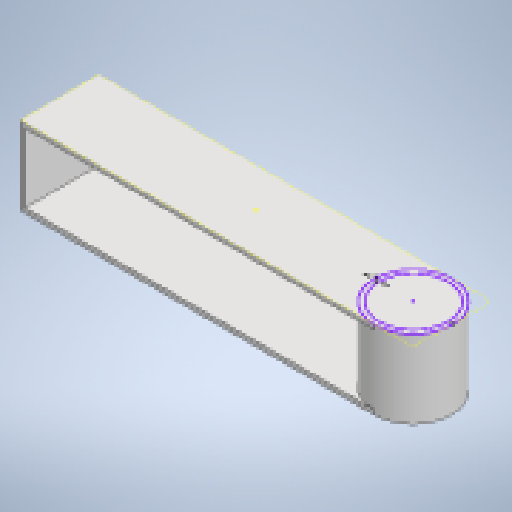
# Autodesk Inventor part: Base_box
Saved by Autodesk Inventor 2023 (Build 270158000, 158)
## iProperties
Created: 2022-04-08
Part Number: Base_box
Material: 一般
Document SubType Name: Modeling
Designer: device
Density: 1 g/cm^3
Appearance: 預設
Author: device
Autodesk Inventor part; units mm, degrees
ref_plane "YZ Plane" through (0, 0, 0) normal (1, 0, 0) x (0, 1, 0)
ref_plane "XZ Plane" through (0, 0, 0) normal (0, 1, 0) x (-1, 0, 0)
ref_plane "XY Plane" through (0, 0, 0) normal (0, 0, 1) x (1, 0, 0)
sketch "草圖1" plane through (0, 0, 0) normal (0, 1, 0) x (-1, 0, 0)
  line L0 (125, 25) -> (-125, 25)
  line L1 (-125, 25) -> (-125, -25)
  line L2 (-125, -25) -> (125, -25)
  line L3 (125, -25) -> (125, 25)
  line L4 (125, 25) -> (-125, -25) construction
  line L5 (-125, 25) -> (125, -25) construction
  point P0 (0, 0)
  dimension "d0" = 250
  dimension "d1" = 50
  constraints: 12 end point, 2 midpoint, 2 parallel, 1 horizontal, 1 perpendicular
  measures "d0" distance of L1.end L2.end
  measures "d1" distance of L0.end L1.end
extrude "擠出1" add sketch "草圖1" along normal blind 50
shell "薄殼1" thickness 3 removed faces 1 at (-41.6667, 16.6667, 25)
sketch "草圖2" plane through (0, 50, 0) normal (0, 1, 0) x (1, 0, 0)
  line L0 (125, -25) -> (125, 25) construction
  line L1 (125, 25) -> (-125, 25) construction
  line L2 (-125, 25) -> (-125, -25) construction
  line L3 (-125, -25) -> (125, -25) construction
  circle A0 centre (100, 0) radius 25
  circle A1 centre (100, 0) radius 22
  point P0 (0, 0)
  point P1 (125, 0)
  dimension "d5" = 3
  constraints: 1 centre point, 1 horizontal, 1 horizontal alignment, 1 midpoint, 2 other
extrude "擠出2" add sketch "草圖2" against normal up to surface (50 mm away)
sketch "草圖4" plane through (0, 50, 0) normal (0, 1, 0) x (1, 0, 0)
  point P0 (0, 0)
sketch "草圖5" plane through (0, 50, 0) normal (0, 1, 0) x (1, 0, 0)
  line L0 (125, 25) -> (-125, 25) construction
  line L1 (-125, 25) -> (-125, -25) construction
  line L2 (-125, -25) -> (125, -25) construction
  line L3 (125, -25) -> (125, 25) construction
  line L4 (125, 0) -> (100, 0) construction
  line L5 (100, 0) -> (100, 25) construction
  line L6 (125, 25) -> (-125, 25) construction
  circle A0 centre (100, 0) radius 35.3553
  point P0 (0, 0)
  constraints: 4 end point, 2 perpendicular, 1 coincident, 1 horizontal, 1 midpoint, 1 point on line, 3 other
extrude "擠出4" cut sketch "草圖5" against normal blind 3
sketch "草圖6" plane through (-122, 47, -22) normal (0, -1, 0) x (1, 0, 0)
  line L0 (210.1257, 0) -> (194.3233, 0) projected
  arc A0 (244, 33.8743) -> (210.1257, 0) centre (222, 22) ccw projected
  line L1 (244, 47) -> (244, 33.8743) projected
  line L2 (247, 47) -> (244, 47) projected
  line L3 (247, -3) -> (247, 47) projected
  line L4 (197, -3) -> (247, -3) projected
  arc A1 (194.3233, 0) -> (197, -3) centre (222, 22) ccw projected
  circle A2 centre (222, 22) radius 22 projected
  arc A3 (233.8743, 0) -> (244, 10.1257) centre (222, 22) ccw projected
  line L5 (244, 0) -> (233.8743, 0) projected
  line L6 (244, 10.1257) -> (244, 0) projected
  arc A4 (197, 47) -> (197, -3) centre (222, 22) ccw projected
  line L7 (197, -3) -> (-3, -3) projected
  line L8 (-3, -3) -> (-3, 47) projected
  line L9 (-3, 47) -> (197, 47) projected
  line L10 (197, 47) -> (244, 47)
  arc A5 (222, 47) -> (210.1257, 0) centre (222, 22) ccw projected
  circle A6 centre (222, 22) radius 38.3553
  point P0 (122, 22)
  point P1 (222, 47)
  point P2 (192.9117, 47)
  point P3 (192.9117, -3)
  point P4 (197, -3)
  dimension "d14" = 3
  constraints: 2 end point, 1 centre point, 1 coincident, 1 perpendicular
  measures "d14" radial gap between concentric circles of A6 A4
extrude "擠出5" add sketch "草圖6" along normal blind 3 contours L0 A4 L10 A0 | A1 L7 A6 L9 A4 | L10 L1 A0 | A3 L6 L5
fillet "圓角1" radius 3 1 edges at (61.6917, 47, 1.8994)
